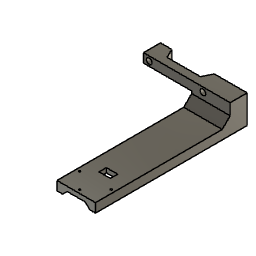
Pan Tilt Small Drone Mount v9 (Autodesk Fusion 360 design; units mm, degrees)
Autodesk Fusion 360 part; units mm, degrees
sketch "Sketch1" plane through (0, 0, 0) normal (0, 1, 0) x (1, 0, 0)
  line L0 (0, 0) -> (67.945, 0)
  line L1 (67.945, 0) -> (67.945, -10.16)
  line L2 (67.945, -10.16) -> (0, -10.16)
  line L3 (0, -10.16) -> (0, 0)
  line L4 (0, -10.16) -> (10.16, -10.16)
  line L5 (10.16, -10.16) -> (10.16, 0)
  line L6 (10.16, 0) -> (0, 0)
  line L7 (0, 0) -> (0, -10.16)
  line L8 (67.945, -10.16) -> (57.785, -10.16)
  line L9 (57.785, -10.16) -> (57.785, 0)
  line L10 (57.785, 0) -> (67.945, 0)
  line L11 (67.945, 0) -> (67.945, -10.16)
  point P0 (3.81, -5.08)
  point P1 (64.135, -5.08)
  dimension "d1" = 60.325
  dimension "d2" = 5.08
  dimension "d3" = 5.08
  dimension "d4" = 3.81
  dimension "d5" = 3.81
  constraint horizontal P0 P1
  constraint horizontal L0
  constraint vertical L1
  constraint horizontal L2
  constraint vertical L3
  constraint coincident L0.start L3.end
  constraint horizontal L4
  constraint vertical L5
  constraint horizontal L6
  constraint vertical L7
  constraint horizontal L8
  constraint vertical L9
  constraint horizontal L10
  constraint vertical L11
  constraint collinear L0 L10
  constraint collinear L0 L6
  constraint equal L8 L9
  constraint equal L5 L6
  measures "d1" distance of P0 P1
  measures "d2" distance of P1 L0
  measures "d3" distance of P1 L2
  measures "d4" distance of P1 L1
  measures "d5" distance of P0 L3
extrude "Extrude1" add sketch "Sketch1" along normal blind 4.064 contours L0 L2 L3 L4 L5 L6 L7 | L0 L1 L2 L8 L9 L10 L11 makes body 1 at (3.3867, 0, 3.3867) makes body 2 at (64.5583, 0, 3.3867)
extrude "Extrude2" add sketch "Sketch1" against normal blind 2.286 bodies 1 2
hole "Hole1" at (64.135, 0, 5.08) at (3.81, 0, 5.08) direction (0, -1, 0) diameter 3.4925 end through all bodies 1
hole "Hole2" at (3.81, 0, 5.08) at (64.135, 0, 5.08) direction (0, 1, 0) diameter 3.4925 end through all bodies 1
sketch "Sketch2" plane through (0, -2.286, 0) normal (0, -1, 0) x (1, 0, 0)
  circle A0 centre (64.135, 5.08) radius 1.7463
  circle A1 centre (3.81, 5.08) radius 1.7463
  line L0 (67.945, 0) -> (67.945, 10.16)
  line L1 (0, 10.16) -> (0, 0)
  line L2 (94.6658, -21.59) -> (94.6658, -11.43)
  line L3 (94.6658, -11.43) -> (51.4858, -11.43)
  line L4 (51.4858, -11.43) -> (51.4858, -21.59)
  line L5 (88.3158, -21.59) -> (88.3158, -16.51)
  line L6 (88.3158, -16.51) -> (57.8358, -16.51)
  line L7 (57.8358, -16.51) -> (57.8358, -21.59)
  line L8 (51.4858, -21.59) -> (57.8358, -21.59)
  line L9 (88.3158, -21.59) -> (94.6658, -21.59)
  line L10 (73.0758, -11.43) -> (73.0758, -16.51)
  line L11 (67.945, 10.16) -> (0, 10.16)
  line L12 (51.4858, -11.43) -> (94.6658, -11.43)
  line L13 (94.6658, -11.43) -> (94.6658, 10.16)
  line L14 (94.6658, 10.16) -> (51.4858, 10.16)
  line L15 (51.4858, 10.16) -> (51.4858, -11.43)
  point P0 (33.9725, 10.16)
  point P1 (73.0758, 10.16)
  dimension "d20" = 21.59
  dimension "d21" = 6.35
  dimension "d28" = 43.18
  dimension "d29" = 39.1033
  dimension "d45" = 10.16
  constraint horizontal L8
  constraint vertical L2
  constraint horizontal L3
  constraint vertical L4
  constraint vertical L5
  constraint horizontal L6
  constraint vertical L7
  constraint collinear L8 L9
  constraint equal L8 L9
  constraint midpoint L3 L10.start
  constraint midpoint L6 L10.end
  constraint equal L5 L10
  constraint horizontal L12
  constraint vertical L13
  constraint horizontal L14
  constraint vertical L15
  constraint coincident L11 L13.end
  constraint collinear L2 L13
  constraint midpoint L11 P0
  constraint midpoint L14 P1
  measures "d20" distance of L3 L11
  measures "d21" distance of L2.start L5.start
  measures "d28" distance of L3.end L2.end
  measures "d29" distance of P0 P1
  measures "d45" distance of L2.start L2.end
extrude "Extrude3" add sketch "Sketch2" along normal blind 6.35 contours A0 | L3 L11 L12 L13 L14 L15 bodies 1
extrude "Extrude4" add sketch "Sketch2" along normal blind 157.48 contours L2 L3 L5 L6 L9 L10 L12 | L3 L4 L6 L7 L8 L10 L12 bodies 1
chamfer "Chamfer1" distance 8.89 angle 45 1 edges at (73.0758, -8.636, -11.43) on bodies 1
extrude "Extrude5" add 1 faces at (67.945, 1.9473, 3.3867) along direction (1, 0, 0) blind 26.7208 on bodies 1 bodies 1
hole "Hole3" at (64.135, 0, 5.08) direction (0, -1, 0) diameter 6.35 end through all bodies 1
extrude "Extrude6" add 1 faces at (36.1743, -2.286, 5.1235) along direction (0, -1, 0) blind 6.35 on bodies 1 bodies 1
hole "Hole4" at (3.81, 0, 5.08) direction (0, -1, 0) diameter 6.35 end through all bodies 1
sketch "Sketch3" plane through (0, 0, -11.43) normal (0, 0, 1) x (-1, 0, 0)
  line L0 (-94.6658, 17.526) -> (-51.4858, 17.526)
  line L1 (-51.4858, 17.526) -> (-51.4858, 159.766)
  line L2 (-51.4858, 159.766) -> (-94.6658, 159.766)
  line L3 (-94.6658, 159.766) -> (-94.6658, 17.526)
  circle A0 centre (-73.0758, 120.6636) radius 1.016
  circle A1 centre (-90.722, 138.3098) radius 1.016
  circle A2 centre (-73.0758, 155.956) radius 1.016
  circle A3 centre (-55.4296, 138.3098) radius 1.016
  line L4 (-73.0758, 121.6796) -> (-73.0758, 154.94)
  line L5 (-56.4456, 138.3098) -> (-89.706, 138.3098)
  line L6 (-51.4858, 138.3098) -> (-55.4296, 138.3098)
  line L7 (-90.722, 138.3098) -> (-94.6658, 138.3098)
  line L8 (-66.7258, 119.6476) -> (-79.4258, 119.6476)
  line L9 (-79.4258, 119.6476) -> (-79.4258, 127.8391)
  line L10 (-79.4258, 127.8391) -> (-66.7258, 127.8391)
  line L11 (-66.7258, 127.8391) -> (-66.7258, 119.6476)
  line L12 (-72.037, 121.6796) -> (-74.1146, 121.6796)
  line L13 (-56.4456, 137.7199) -> (-56.4456, 138.8996)
  point P0 (-73.0758, 127.8391)
  point P1 (-73.0758, 121.6796)
  point P2 (-56.4456, 138.3098)
  dimension "d39" = 2.032
  dimension "d40" = 24.9555
  dimension "d41" = 24.9555
  dimension "d42" = 24.9555
  dimension "d43" = 3.81
  dimension "d49" = 12.7
  dimension "d54" = 7.1755
  constraint vertical A0.centre A2.centre
  constraint horizontal A1.centre A3.centre
  constraint equal A0 A1
  constraint equal A0 A3
  constraint equal A0 A2
  constraint coincident A0 P1
  constraint vertical L4
  constraint coincident A3 P2
  constraint coincident A1 L5.end
  constraint horizontal L5
  constraint equal L4 L5
  constraint coincident A2 L4.end
  constraint coincident L1 L6.start
  constraint coincident A3.centre L6.end
  constraint horizontal L6
  constraint coincident A1.centre L7.start
  constraint coincident L3 L7.end
  constraint perpendicular L3 L7
  constraint equal L6 L7
  constraint horizontal L8
  constraint vertical L9
  constraint horizontal L10
  constraint vertical L11
  constraint midpoint L10 P0
  constraint coincident L4 P0
  constraint horizontal L12
  constraint coincident P1 L12
  constraint midpoint L12 P1
  constraint coincident L4 P1
  constraint tangent A0 L12
  constraint vertical L13
  constraint midpoint L13 P2
  constraint coincident L5 P2
  constraint tangent A3 L13
  constraint tangent A0 L8
  measures "d39" diameter of A0
  measures "d40" distance of A0.centre A1.centre
  measures "d41" distance of A0.centre A3.centre
  measures "d42" distance of A1.centre A2.centre
  measures "d43" distance of L2 A2.centre
  measures "d49" distance of L9.end L10.end
  measures "d54" distance of A0.centre L10
extrude "Extrude7" cut sketch "Sketch3" against normal through all contours A1 | A3 | A0 | A0 L4 L8 L10 L11 | A0 L4 L8 L9 L10 | A2 bodies 1
ref_plane "WorkPlane1" through (73.0758, -84.201, -15.24) normal (0, 0, 1) x (-1, 0, 0)
sketch "Sketch4" plane through (0, 0, -15.24) normal (0, 0, 1) x (1, 0, 0)
  circle A0 centre (55.4296, -138.3098) radius 1.778
  circle A1 centre (73.0758, -155.956) radius 1.778
  circle A2 centre (90.722, -138.3098) radius 1.778
  circle A3 centre (55.4296, -138.3098) radius 1.016
  circle A4 centre (73.0758, -155.956) radius 1.016
  circle A5 centre (90.722, -138.3098) radius 1.016
  dimension "d47" = 3.556
  constraint concentric A0 A3
  constraint concentric A1 A4
  constraint concentric A2 A5
  constraint equal A1 A2
  constraint equal A0 A1
  measures "d47" diameter of A1
extrude "Extrude8" cut sketch "Sketch4" against normal through all contours A0 | A1 | A2 | A3 | A4 | A5 bodies 1
chamfer "Chamfer3" distance 5.08 angle 45 2 edges at (57.8358, -81.026, -16.51) (88.3158, -81.026, -16.51) on bodies 1
extrude "Extrude10" add 2 faces at (85.0693, 4.064, 5.1235) (8.6238, 4.064, 5.1235) along direction (0, 1, 0) blind 6.35 on bodies 1 bodies 1
extrude "Extrude11" add 1 faces at (0, -2.286, 3.3867) along direction (-1, 0, 0) blind 2.54 on bodies 1 bodies 1
extrude "Extrude12" add 1 faces at (76.4628, -2.286, -5.5033) along direction (0, 1, 0) blind 2.286 on bodies 1 bodies 1
sketch "Sketch5" plane through (0, 0, 0) normal (0, 1, 0) x (-1, 0, 0)
  line L0 (-10.16, 0) -> (-10.16, 10.16)
  line L1 (-10.16, 10.16) -> (-57.785, 10.16)
  line L2 (-57.785, 10.16) -> (-57.785, 0)
  line L3 (-57.785, 0) -> (-94.6658, 0)
  line L4 (-94.6658, 0) -> (-94.6658, -21.59)
  line L5 (-94.6658, -21.59) -> (-88.3158, -21.59)
  line L6 (-88.3158, -21.59) -> (-83.2358, -16.51)
  line L7 (-83.2358, -16.51) -> (-62.9158, -16.51)
  line L8 (-62.9158, -16.51) -> (-57.8358, -21.59)
  line L9 (-57.8358, -21.59) -> (-51.4858, -21.59)
  line L10 (-51.4858, -21.59) -> (-51.4858, 0)
  line L11 (-51.4858, 0) -> (-10.16, 0)
  line L12 (-57.785, 0) -> (-51.4858, 0)
  constraint coincident L2.end L3.start
  constraint coincident L10.end L11.start
extrude "Extrude13" add sketch "Sketch5" along normal blind 10.414 contours L3 L4 L5 L6 L7 L8 L9 L10 L12 bodies 1
chamfer "Chamfer5" distance 10.414 distance2 5.08 1 edges at (10.16, 0, 5.08) measured on face at (10.16, 3.4713, 6.7733) on bodies 1
chamfer "Chamfer5" distance 5.08 distance2 10.414 1 edges at (57.785, 0, 5.08) measured on face at (39.8103, 0, 6.7733) on bodies 1
equation "d12 = -0.25 in + 0.16 in"
equation "d20 = 0.55 in + 0.2 in + 0.1 in"
equation "d40 = 1.0575 in - 0.075 in"
equation "d41 = 1.0575 in - 0.075 in"
equation "d42 = 1.0575 in - 0.075 in"
